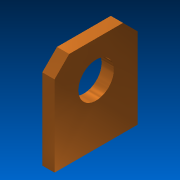
# Autodesk Inventor part: Omron SS-01GL2-E Microswitch Contact
Saved by Autodesk Inventor 2016 (Build 200138000, 138)
## iProperties
Created: 2012-05-23
Material: Gold
Document SubType Name: Modeling
Designer: sdarley
Density: 1 g/cm^3
Project: Microswitch - Omron SS-01GL2-E
Description: Omron SS-01GL2-E Microswitch Contact
Appearance: Metal 1600F Hot
Author: sdarley
Title: Omron SS-01GL2-E Microswitch Contact
Revision Number: 1
Autodesk Inventor part; units mm, degrees
ref_plane "YZ Plane" through (0, 0, 0) normal (1, 0, 0) x (0, 1, 0)
ref_plane "XZ Plane" through (0, 0, 0) normal (0, 1, 0) x (-1, 0, 0)
ref_plane "XY Plane" through (0, 0, 0) normal (0, 0, 1) x (1, 0, 0)
sketch "Sketch1" plane through (0, 0, 0) normal (1, 0, 0) x (0, 1, 0)
  line L0 (1.7, 0) -> (-1.7, 0)
  line L1 (-1.7, 0) -> (-1.7, 3.9)
  line L2 (-1.7, 3.9) -> (1.7, 3.9)
  line L3 (1.7, 3.9) -> (1.7, 0)
  circle A0 centre (0, 2.425) radius 0.725
  point P0 (0, 0)
  point P1 (0, 0)
  dimension "d0" = 3.9
  dimension "d2" = 3.4
  dimension "d3" = 1.45
  dimension "d4" = 0.75
  constraints: 8 end point, 2 coincident, 2 parallel, 1 centre point, 1 horizontal, 1 midpoint, 1 perpendicular, 1 vertical alignment
  measures "d0" distance of L0.end L1.end
  measures "d2" distance of L1.end L2.end
  measures "d3" diameter of A0
  measures "d4" distance edge to line of A0 L2
extrude "Extrusion1" add sketch "Sketch1" along normal blind 0.5
chamfer "Chamfer1" distance 0.6 angle 45 2 edges at (0.25, 1.7, 3.9) (0.25, -1.7, 3.9)
body "Solid1"
